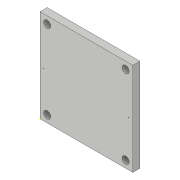
# Autodesk Inventor part: STAND PLATE FOR STORSGE SYSTEM
Saved by Autodesk Inventor 2019 (Build 230136000, 136)
## iProperties
Created: 2019-10-14
Part Number: STAND PLATE FOR STORSGE SYSTEM
Material: Generic
Document SubType Name: Modeling
Designer: Admin
Density: 1 g/cm^3
Appearance: Default
Author: Admin
Autodesk Inventor part; units mm, degrees
ref_plane "YZ Plane" through (0, 0, 0) normal (1, 0, 0) x (0, 1, 0)
ref_plane "XZ Plane" through (0, 0, 0) normal (0, 1, 0) x (-1, 0, 0)
ref_plane "XY Plane" through (0, 0, 0) normal (0, 0, 1) x (1, 0, 0)
sketch "Sketch1" plane through (0, 0, 0) normal (0, 0, 1) x (1, 0, 0)
  line L0 (0, 0) -> (130, 0)
  line L1 (130, 0) -> (130, 130)
  line L2 (130, 130) -> (0, 130)
  line L3 (0, 130) -> (0, 0)
  dimension "d0" = 130
  dimension "d1" = 130
  constraints: 8 end point, 2 parallel, 1 horizontal, 1 perpendicular
  measures "d0" distance of L2.end L1.end
  measures "d1" distance of L1.end L0.end
extrude "Extrusion1" add sketch "Sketch1" along normal blind 10
sketch "Sketch2" plane through (0, 0, 10) normal (0, 0, 1) x (1, 0, 0)
  line L0 (0, 0) -> (130, 0) projected
  line L1 (0, 0) -> (10, 0)
  line L2 (10, 0) -> (10, 110)
  line L3 (10, 110) -> (10, 120)
  line L4 (10, 120) -> (120, 120)
  line L5 (120, 120) -> (120, 10)
  line L6 (120, 10) -> (10, 10)
  circle A0 centre (10, 120) radius 5
  circle A1 centre (120, 120) radius 5
  circle A2 centre (10, 10) radius 5
  circle A3 centre (120, 10) radius 5
  dimension "d4" = 10
  dimension "d5" = 110
  dimension "d6" = 10
  dimension "d7" = 110
  dimension "d8" = 110
  dimension "d9" = 110
  dimension "d10" = 10
  dimension "d11" = 10
  dimension "d12" = 10
  dimension "d13" = 10
  constraints: 12 end point, 4 centre point, 4 coincident, 3 perpendicular, 3 point on line
  measures "d4" distance of L0.start L1.end
  measures "d5" distance of L1.end L2.end
  measures "d6" distance of L2.end L3.end
  measures "d7" distance of L3.end L4.end
  measures "d8" distance of L4.end L5.end
  measures "d9" distance of L5.end L6.end
  measures "d10" diameter of A0
  measures "d11" diameter of A1
  measures "d12" diameter of A2
  measures "d13" diameter of A3
extrude "Extrusion2" cut sketch "Sketch2" against normal through all contours A2 L2 | L2 L6 A2 | L2 A2 L6 | A3 L5 L6 | L6 L5 A3 | A0 L4 L3 | L3 L4 A0 | A1 L4 L5 | L5 L4 A1
sketch "Sketch3" plane through (0, 0, 10) normal (0, 0, 1) x (1, 0, 0)
  line L0 (0, 0) -> (130, 0) projected
  line L1 (68.2625, 0) -> (63.2625, 0)
  line L2 (63.2625, 0) -> (63.2625, 5)
  circle A0 centre (63.2625, 5) radius 0.05
  dimension "d16" = 5
  dimension "d17" = 5
  dimension "d18" = 0.1
  constraints: 4 end point, 2 point on line, 1 centre point, 1 coincident, 1 perpendicular
  measures "d16" distance of L1.start L1.end
  measures "d17" distance of L1.end L2.end
  measures "d18" diameter of A0
extrude "Extrusion3" cut sketch "Sketch3" along normal through all both and the other way through all
sketch "Sketch4" plane through (0, 0, 10) normal (0, 0, 1) x (1, 0, 0)
  line L0 (63.5, 131.7625) -> (63.5, 126.7625)
  circle A0 centre (63.5, 126.7625) radius 0.05
  point P0 (0, 0)
  dimension "d21" = 5
  dimension "d22" = 0.1
  constraints: 2 end point, 1 centre point, 1 coincident, 1 vertical
  measures "d21" distance of L0.start L0.end
  measures "d22" diameter of A0
extrude "Extrusion4" cut sketch "Sketch4" against normal blind 10
sketch "Sketch5" plane through (0, 0, 10) normal (0, 0, 1) x (1, 0, 0)
  line L0 (0, 63.5) -> (5, 63.5)
  line L1 (5, 63.5) -> (123.825, 63.5)
  circle A0 centre (5, 63.5) radius 0.5
  circle A1 centre (123.825, 63.5) radius 0.5
  point P0 (0, 0)
  dimension "d25" = 5
  dimension "d26" = 1
  dimension "d27" = 1
  constraints: 4 end point, 2 centre point, 2 coincident, 1 horizontal, 1 point on line
  measures "d25" distance of L0.start L0.end
  measures "d26" diameter of A0
  measures "d27" diameter of A1
extrude "Extrusion5" cut sketch "Sketch5" against normal through all
sketch "Sketch6" plane through (0, 0, 10) normal (0, 0, 1) x (1, 0, 0)
  point P0 (0, 0)
body "Solid1"
